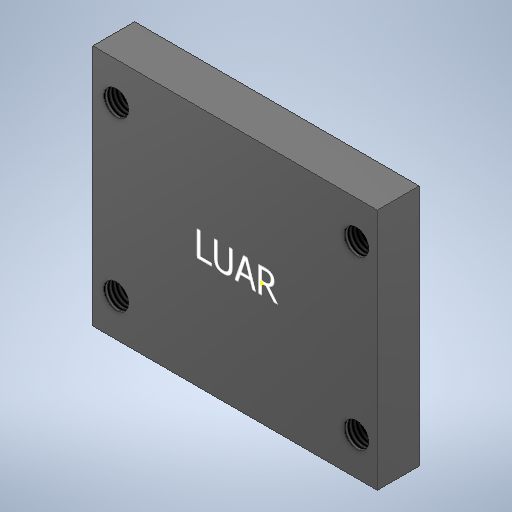
# Autodesk Inventor part: Part1
Saved by Autodesk Inventor 2025.1 (Build 291241000, 241)
## iProperties
Created: 2024-09-21
Part Number: Part1
Material: ABS Plastic
Document SubType Name: Modeling
Designer: JuhenFW
Density: 1.06 g/cm^3
Appearance: Smooth - White
Author: JuhenFW
Autodesk Inventor part; units mm, degrees
ref_plane "YZ Plane" through (0, 0, 0) normal (1, 0, 0) x (0, 1, 0)
ref_plane "XZ Plane" through (0, 0, 0) normal (0, 1, 0) x (-1, 0, 0)
ref_plane "XY Plane" through (0, 0, 0) normal (0, 0, 1) x (1, 0, 0)
sketch "Sketch1" plane through (0, 0, 0) normal (0, 0, 1) x (1, 0, 0)
  line L0 (-20.1958, -14.566) -> (13.8042, -14.566)
  line L1 (13.8042, -14.566) -> (13.8042, 14.434)
  line L2 (13.8042, 14.434) -> (-20.1958, 14.434)
  line L3 (-20.1958, 14.434) -> (-20.1958, -14.566)
  circle A0 centre (11.3042, 9.934) radius 1.5
  circle A1 centre (11.3042, -10.066) radius 1.5
  circle A2 centre (-17.3958, 9.934) radius 1.5
  circle A3 centre (-17.3958, -10.066) radius 1.5
  point P0 (0, 0)
  dimension "d1" = 34
  dimension "d2" = 3
  dimension "d3" = 3
  dimension "d4" = 20
  dimension "d5" = 3
  dimension "d6" = 3
  dimension "d8" = 28.7
  dimension "d9" = 2.5
  dimension "d10" = 20
  dimension "d11" = 29
  dimension "d12" = 4.5
  constraints: 8 end point, 4 centre point, 2 horizontal alignment, 2 parallel, 1 horizontal, 1 perpendicular, 1 vertical alignment
  measures "d1" distance between parallel lines of L1 L3
  measures "d2" diameter of A0
  measures "d3" diameter of A1
  measures "d4" distance of A1.centre A0.centre
  measures "d5" diameter of A2
  measures "d6" diameter of A3
  measures "d8" distance of A0.centre A2.centre
  measures "d9" distance from line of L1 A1.centre
  measures "d10" distance of A3.centre A2.centre
  measures "d11" distance between parallel lines of L0 L2
  measures "d12" distance from line of L2 A0.centre
extrude "Extrusion1" add sketch "Sketch1" along normal blind 5
thread "Thread1" size "M3x0.5" class "6H" standard "ANSI Metric M Profile" length 5
thread "Thread2" size "M3x0.5" class "6H" standard "ANSI Metric M Profile" length 5
thread "Thread3" size "M3x0.5" class "6H" standard "ANSI Metric M Profile" length 5
thread "Thread4" size "M3x0.5" class "6H" standard "ANSI Metric M Profile" length 5
sketch "Sketch3" plane through (0, 0, 5) normal (0, 0, 1) x (1, 0, 0)
  line L0 (-9.0293, 4.1042) -> (2.8565, 4.1042) construction
  line L1 (2.8565, 4.1042) -> (2.8565, -3.7102) construction
  line L2 (2.8565, -3.7102) -> (-9.0293, -3.7102) construction
  line L3 (-9.0293, -3.7102) -> (-9.0293, 4.1042) construction
  point P0 (0, 0)
  dimension "d3" = 3
  constraints: 2 other
body "Solid1"
